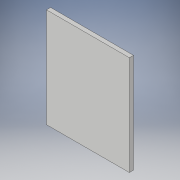
# Autodesk Inventor part: Chassis-2
Saved by Autodesk Inventor 2018 (Build 220112000, 112)
## iProperties
Created: 2018-01-20
Part Number: Chassis-2
Material: Generisch
Document SubType Name: Modeling
Designer: fhinstall
Density: 1 g/cm^3
Appearance: Vorgabe
Author: fhinstall
Autodesk Inventor part; units mm, degrees
ref_plane "YZ Plane" through (0, 0, 0) normal (1, 0, 0) x (0, 1, 0)
ref_plane "XZ Plane" through (0, 0, 0) normal (0, 1, 0) x (-1, 0, 0)
ref_plane "XY Plane" through (0, 0, 0) normal (0, 0, 1) x (1, 0, 0)
sketch "Skizze1" plane through (0, 0, 0) normal (0, 1, 0) x (-1, 0, 0)
  line L0 (50, 60) -> (50, -60)
  line L1 (50, -60) -> (-50, -60)
  line L2 (-50, -60) -> (-50, 60)
  line L3 (-50, 60) -> (50, 60)
  line L4 (0, 61.8387) -> (0, -63.7479) construction
  line L5 (83.0665, 0) -> (-88.5254, 0) construction
  point P0 (0, 0)
  dimension "d1" = 50
  dimension "d2" = 50
  dimension "d3" = 60
  dimension "d4" = 60
  constraints: 12 end point, 2 perpendicular, 2 point on line, 2 vertical, 1 horizontal
  measures "d1" distance between parallel lines of L0 L4
  measures "d2" distance between parallel lines of L2 L4
  measures "d3" distance between parallel lines of L5 L3
  measures "d4" distance between parallel lines of L5 L1
extrude "Extrusion1" add sketch "Skizze1" along normal blind 5
